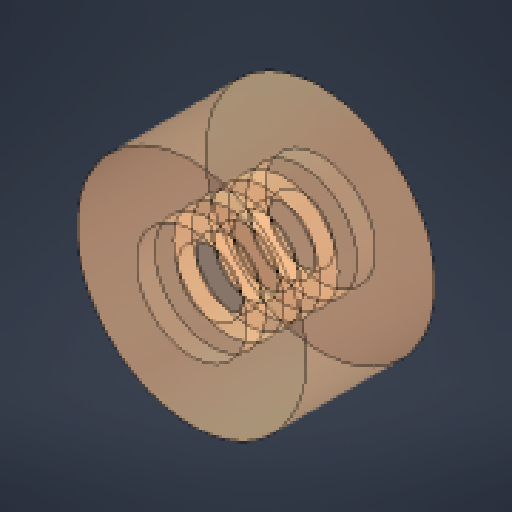
# Autodesk Inventor part: opona
Saved by Autodesk Inventor 2023 (Build 270158000, 158)
## iProperties
Created: 2024-03-01
Part Number: opona
Material: Rubber, Silicone
Document SubType Name: Modeling
Designer: Michał
Density: 1.25 g/cm^3
Appearance: Rubber - Black
Author: Michał
Autodesk Inventor part; units mm, degrees
ref_plane "YZ Plane" through (0, 0, 0) normal (1, 0, 0) x (0, 1, 0)
ref_plane "XZ Plane" through (0, 0, 0) normal (0, 1, 0) x (-1, 0, 0)
ref_plane "XY Plane" through (0, 0, 0) normal (0, 0, 1) x (1, 0, 0)
sketch "Sketch1" plane through (0, 0, 0) normal (1, 0, 0) x (0, 1, 0)
  line L0 (3.5, -4) -> (3.5, -2)
  line L1 (6, -2) -> (6, 0)
  line L2 (6, -6) -> (6, -4)
  line L3 (3.5, -8) -> (3.5, -6)
  line L4 (6, -10) -> (6, -8)
  line L5 (3.4951, -12) -> (3.4951, -10) projected
  line L6 (6, -14) -> (6, -12)
  line L7 (0, 0) -> (0, -14)
  line L8 (6, 0) -> (12.5, 0)
  line L9 (12.5, 0) -> (12.5, -14)
  line L10 (12.5, -14) -> (6, -14)
  line L11 (6, -12) -> (3.4951, -12)
  line L12 (3.4951, -10) -> (6, -10)
  line L13 (6, -8) -> (3.5, -8)
  line L14 (3.5, -6) -> (6, -6)
  line L15 (6, -4) -> (3.5, -4)
  line L16 (3.5, -2) -> (6, -2)
  point P0 (9.25, 0)
  dimension "d1" = 12.5
  constraints: 32 end point, 8 vertical, 5 parallel, 2 horizontal, 1 coincident, 1 horizontal alignment, 1 midpoint, 1 perpendicular, 12 other
  measures "d1" distance between parallel lines of L9 L7
revolve "Revolution1" add sketch "Sketch1" angle 360 about axis through (0, 0, 0) along (0, 0, -1)
sketch "Sketch2" plane through (0, 0, 0) normal (0, 0, 1) x (1, 0, 0)
  circle A0 centre (-0.9457, -4.1434) radius 1 projected
  circle A1 centre (-3.8291, 1.844) radius 1 projected
  circle A2 centre (2.6498, 3.3228) radius 1 projected
  circle A3 centre (4.25, 0) radius 1 projected
  circle A4 centre (-0.9457, 4.1434) radius 1 projected
  circle A5 centre (-3.8291, -1.844) radius 1 projected
  circle A6 centre (2.6498, -3.3228) radius 1 projected
  circle A7 centre (0, 0) radius 6 projected
  point P0 (0, 0)
extrude "Extrusion1" add sketch "Sketch2" against normal up to surface (14 mm away) contours A0 | A1 | A2 | A3 | A4 | A5 | A6
body "Solid1"
